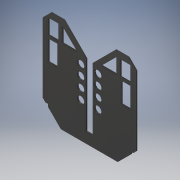
# Autodesk Inventor part: Kermit Board
Saved by Autodesk Inventor 2018.2 (Build 222227000, 227)
## iProperties
Created: 2018-02-17
Part Number: Kermit Board
Material: Glass
Document SubType Name: Modeling
Designer: lopez.xavier
Density: 2.18 g/cm^3
Appearance: Dark Gray
Author: lopez.xavier
Autodesk Inventor part; units mm, degrees
ref_plane "YZ Plane" through (0, 0, 0) normal (1, 0, 0) x (0, 1, 0)
ref_plane "XZ Plane" through (0, 0, 0) normal (0, 1, 0) x (-1, 0, 0)
sketch "Sketch1" plane through (0, 0, 0) normal (0, 0, 1) x (1, 0, 0)
  line L0 (0, 0) -> (228.6, 0)
  line L1 (228.6, 0) -> (228.6, 469.9)
  line L2 (228.6, 469.9) -> (0, 469.9)
  line L3 (0, 469.9) -> (0, 0)
  dimension "d0" = 469.9
  dimension "d1" = 228.6
  constraints: 8 end point, 2 parallel, 1 horizontal, 1 perpendicular
  measures "d0" distance of L0.end L1.end
  measures "d1" distance of L1.end L2.end
extrude "Extrusion1" add sketch "Sketch1" along normal blind 6.35
sketch "Sketch2" plane through (0, 0, 6.35) normal (0, 0, 1) x (1, 0, 0)
  line L0 (228.6, 469.9) -> (0, 469.9) projected
  line L1 (38.1, 469.9) -> (0, 431.8)
  line L2 (0, 469.9) -> (0, 0) projected
  line L3 (0, 88.9) -> (88.9, 0)
  line L4 (0, 0) -> (228.6, 0) projected
  line L5 (0, 88.9) -> (0, 0)
  line L6 (0, 0) -> (88.9, 0)
  line L7 (38.1, 469.9) -> (0, 469.9)
  line L8 (0, 431.8) -> (0, 469.9)
  circle A0 centre (12.7, 457.2) radius 2.54
  circle A1 centre (12.7, 431.8) radius 2.54
  circle A2 centre (12.7, 406.4) radius 2.54
  circle A3 centre (12.7, 381) radius 2.54
  circle A4 centre (12.7, 355.6) radius 2.54
  circle A5 centre (12.7, 330.2) radius 2.54
  circle A6 centre (12.7, 304.8) radius 2.54
  circle A7 centre (12.7, 279.4) radius 2.54
  circle A8 centre (12.7, 254) radius 2.54
  circle A9 centre (12.7, 228.6) radius 2.54
  circle A10 centre (12.7, 203.2) radius 2.54
  circle A11 centre (12.7, 177.8) radius 2.54
  circle A12 centre (12.7, 152.4) radius 2.54
  circle A13 centre (12.7, 127) radius 2.54
  circle A14 centre (12.7, 101.6) radius 2.54
  circle A15 centre (12.7, 76.2) radius 2.54
  circle A16 centre (12.7, 50.8) radius 2.54
  circle A17 centre (12.7, 25.4) radius 2.54
  line L9 (25.4, 444.5) -> (76.2, 444.5)
  line L10 (76.2, 444.5) -> (76.2, 368.3)
  line L11 (76.2, 368.3) -> (25.4, 368.3)
  line L12 (25.4, 368.3) -> (25.4, 444.5)
  line L13 (25.4, 355.6) -> (71.12, 355.6)
  line L14 (71.12, 355.6) -> (71.12, 254)
  line L15 (71.12, 254) -> (25.4, 254)
  line L16 (25.4, 254) -> (25.4, 355.6)
  line L17 (95.25, 444.5) -> (95.25, 368.3)
  line L18 (95.25, 368.3) -> (171.45, 368.3)
  line L19 (95.25, 444.5) -> (171.45, 368.3)
  line L20 (211.9249, 469.9) -> (211.9249, 50.8)
  line L21 (228.6, 0) -> (228.6, 469.9) projected
  line L22 (101.6, 469.9) -> (228.6, 342.9)
  line L23 (101.6, 469.9) -> (228.6, 469.9)
  line L24 (228.6, 469.9) -> (228.6, 342.9)
  line L25 (211.9249, 50.8) -> (228.6, 50.8)
  line L26 (228.6, 50.8) -> (228.6, 342.9)
  circle A18 centre (186.5249, 325.12) radius 17.78
  circle A19 centre (186.5249, 274.32) radius 17.78
  circle A20 centre (186.5249, 223.52) radius 17.78
  circle A21 centre (186.5249, 172.72) radius 17.78
  line L27 (211.9249, 359.5751) -> (228.6, 342.9)
  line L28 (211.9249, 359.5751) -> (211.9249, 50.8)
  line L29 (211.9249, 50.8) -> (228.6, 50.8)
  line L30 (228.6, 50.8) -> (228.6, 342.9)
  dimension "d4" = 38.1
  dimension "d5" = 38.1
  dimension "d6" = 88.9
  dimension "d7" = 0
  dimension "d8" = 88.9
  dimension "d9" = 5.08
  dimension "d10" = 12.7
  dimension "d11" = 12.7
  dimension "d14" = 25.4
  dimension "d20" = 50.8
  dimension "d21" = 76.2
  dimension "d22" = 25.4
  dimension "d23" = 25.4
  dimension "d24" = 45.72
  dimension "d25" = 101.6
  dimension "d27" = 25.4
  dimension "d28" = 19.05
  dimension "d29" = 76.2
  dimension "d30" = 76.2
  dimension "d31" = 0
  dimension "d32" = 12.7
  dimension "d33" = 16.6751
  dimension "d34" = 0
  dimension "d35" = 50.8
  dimension "d37" = 127
  dimension "d38" = 35.56
  dimension "d39" = 17.78
  dimension "d42" = 50.8
  dimension "d47" = 25.4
  constraints: 54 end point, 22 centre point, 9 point on line, 5 collinear, 5 parallel, 5 perpendicular, 4 horizontal, 4 vertical, 40 other
  measures "d4" distance of L0.end L1.start
  measures "d5" distance of L0.end L1.end
  measures "d6" distance of L2.end L3.start
  measures "d7" distance from line of L4 L3.end
  measures "d8" distance of L2.end L3.end
  measures "d9" diameter of A0
  measures "d10" distance from line of L0 A0.centre
  measures "d11" distance from line of L2 A0.centre
  measures "d14" distance of A0.centre A1.centre
  measures "d20" distance of L10.end L11.end
  measures "d21" distance of L9.end L10.end
  measures "d22" distance between parallel lines of L0 L9
  measures "d23" distance between parallel lines of L2 L12
  measures "d24" distance of L14.end L15.end
  measures "d25" distance of L13.end L14.end
  measures "d27" distance between parallel lines of L2 L16
  measures "d28" distance between parallel lines of L10 L17
  measures "d29" distance of L17.end L18.end
  measures "d30" distance of L17.start L17.end
  measures "d31" distance from line of L9 L17.start
  measures "d32" distance between parallel lines of L11 L13
  measures "d33" distance between parallel lines of L21 L20
  measures "d34" distance from line of L0 L20.start
  measures "d35" distance from line of L4 L20.end
  measures "d37" distance of L0.start L22.end
  measures "d38" diameter of A18
  measures "d39" vertical distance of L22.end A18.centre
  measures "d42" distance of A18.centre A19.centre
  measures "d47" distance from line of L20 A18.centre
extrude "Extrusion2" cut sketch "Sketch2" against normal blind 25.4 contours L21 L22 L20 L0 | L20 L22 L0 | L21 L25 L20 L22 | L1 L2 L0 | L4 L2 L3 A15 | A15 L3 | A0 | A1 | A2 | A3 | A4 | A5 | A6 | A7 | A8 | A9 | A10 | A11 | A12 | A13 | A14 | A16 | A17 | L9 L10 L11 L12 | L13 L14 L15 L16 | L19 L18 L17 | A18 | A19 | A20 | A21 picked at (11.9754, 76.638)
ref_plane "Work Plane2" through (228.6, 0, 6.35) normal (1, 0, 0) x (0, 0, -1)
mirror "Mirror1" about plane through (228.6, 0, 6.35) normal (1, 0, 0) of "Extrusion1", "Extrusion2"
sketch "Sketch3" plane through (0, 0, 6.35) normal (0, 0, 1) x (1, 0, 0)
  circle A0 centre (12.7, 76.2) radius 2.54
  circle A1 centre (12.7, 101.6) radius 2.54 projected
  line L0 (12.7, 76.2) -> (25.4, 76.2)
  line L1 (25.4, 76.2) -> (25.4, 63.5)
  line L2 (88.9, 0) -> (0, 88.9) projected
  line L3 (25.4, 63.5) -> (12.7, 76.2)
  circle A2 centre (444.5, 76.2) radius 2.54
  circle A3 centre (444.5, 101.6) radius 2.54 projected
  line L4 (444.5, 76.2) -> (431.8, 76.2)
  line L5 (431.8, 76.2) -> (431.8, 63.5)
  line L6 (431.8, 63.5) -> (444.5, 76.2)
  line L7 (457.2, 88.9) -> (368.3, 0) projected
  point P0 (0, 0)
  dimension "d52" = 5.08
  dimension "d53" = 25.4
  dimension "d54" = 0
  dimension "d55" = 12.7
  dimension "d56" = 5.08
  dimension "d57" = 25.4
  dimension "d58" = 0
  dimension "d59" = 12.7
  constraints: 12 end point, 2 centre point, 2 horizontal, 2 perpendicular, 1 collinear, 1 point on line
  measures "d52" diameter of A0
  measures "d53" distance of A1.centre L0.start
  measures "d54" horizontal distance of A1.centre L0.start
  measures "d55" distance of L0.start L0.end
  measures "d56" diameter of A2
  measures "d57" distance of A3.centre L4.start
  measures "d58" horizontal distance of A3.centre L4.start
  measures "d59" distance of L4.start L4.end
extrude "Extrusion3" cut sketch "Sketch3" against normal blind 25.4 contours L0 L1 L2 A0 | A0 L2 L0 | L6 L5 L4 A2 | A2 L4 L6 picked at (14.3126, 75.7108)
equation "\"d27\" = d23"
body "Solid1"
